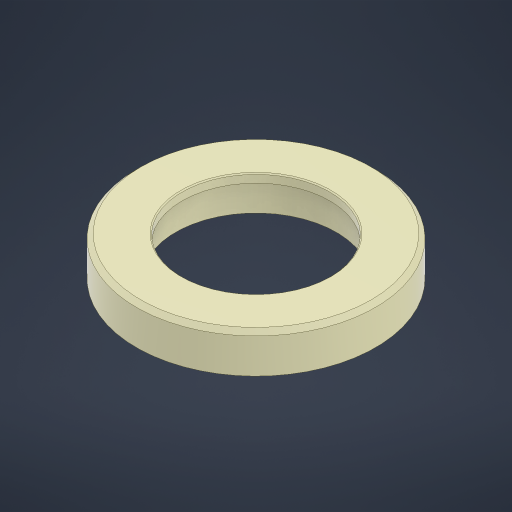
# Autodesk Inventor part: Bearing_Holder
Saved by Autodesk Inventor 2023 (Build 270158000, 158)
## iProperties
Created: 2023-02-16
Part Number: Bearing_Holder
Material: ABS Plastic
Document SubType Name: Modeling
Designer: dzw04
Density: 1.06 g/cm^3
Appearance: Smooth - Ash
Author: dzw04
Autodesk Inventor part; units mm, degrees
ref_plane "YZ Plane" through (0, 0, 0) normal (1, 0, 0) x (0, 1, 0)
ref_plane "XZ Plane" through (0, 0, 0) normal (0, 1, 0) x (-1, 0, 0)
ref_plane "XY Plane" through (0, 0, 0) normal (0, 0, 1) x (1, 0, 0)
sketch "Sketch1" plane through (0, 0, 0) normal (0, 1, 0) x (-1, 0, 0)
  circle A0 centre (0, 0) radius 27.5
  dimension "d0" = 55
  constraints: 1 centre point, 1 coincident
  measures "d0" diameter of A0
extrude "Extrusion1" add sketch "Sketch1" along normal blind 9
sketch "Sketch2" plane through (0, 9, 0) normal (0, 1, 0) x (1, 0, 0)
  circle A0 centre (0, 0) radius 17
  dimension "d3" = 34
  constraints: 1 centre point, 1 coincident
  measures "d3" diameter of A0
extrude "Extrusion2" cut sketch "Sketch2" against normal through all
sketch "Sketch3" plane through (0, 0, 0) normal (0, -1, 0) x (1, 0, 0)
  circle A0 centre (0, 0) radius 18.5
  dimension "d6" = 37
  constraints: 1 centre point, 1 coincident
  measures "d6" diameter of A0
extrude "Extrusion3" cut sketch "Sketch3" against normal blind 7
chamfer "Chamfer1" distance 1 angle 45 1 edges at (27.5, 9, 0)
sketch "Sketch4" plane through (0, 0, 0) normal (0, -1, 0) x (1, 0, 0)
  line L0 (0, 0) -> (0, 22)
  circle A0 centre (0, 22) radius 2.125
  circle A1 centre (-19.0526, -11) radius 2.125
  circle A2 centre (19.0526, -11) radius 2.125
  dimension "d12" = 22
  dimension "d13" = 4.25
  dimension "d16" = 360
  constraints: 3 centre point, 2 end point, 1 coincident, 1 vertical, 7 other
  measures "d12" distance of L0.start L0.end
  measures "d13" diameter of A0
extrude "Extrusion4" cut sketch "Sketch4" against normal blind 6.5
chamfer "Chamfer3" distance 0.25 angle 45 1 edges at (-17, 9, 0)
sketch "Sketch5" plane through (0, 0, 0) normal (0, -1, 0) x (1, 0, 0)
  circle A0 centre (0, 22) radius 2.125 projected
  circle A1 centre (0, 22) radius 3
  circle A2 centre (19.0526, -11) radius 2.125 projected
  circle A3 centre (19.0526, -11) radius 3
  circle A4 centre (-19.0526, -11) radius 2.125 projected
  circle A5 centre (-19.0526, -11) radius 3
  point P0 (0, 0)
  dimension "d26" = 6
  dimension "d27" = 6
  dimension "d28" = 6
  constraints: 3 centre point, 3 coincident
  measures "d26" diameter of A1
  measures "d27" diameter of A3
  measures "d28" diameter of A5
extrude "Extrusion5" cut sketch "Sketch5" against normal blind 1 contours A1 | A2 | A3 | A4 | A5
chamfer "Chamfer7" distance 0.25 angle 45 3 edges at (-2.125, 1, 22) (16.9276, 1, -11) (-21.1776, 1, -11)
body "Solid1"
